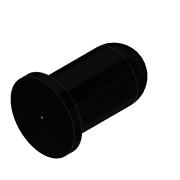
# Autodesk Inventor part: Photodiodendummie
Saved by Autodesk Inventor 2018.2 (Build 222227000, 227)
## iProperties
Created: 2018-10-30
Part Number: Photodiodendummie
Material: Kst - PEEK GF30
Document SubType Name: Modeling
Designer: N.Grubert
Density: 1.49 g/cm^3
Appearance: Grau (Schiefer)
Fläche: 0 cm²
Gewicht: 0 g
Material: geeigneten Werkstoff auswählen !
Dateiname: P:\INVENTOR\Inventor 2018\Templates\ILT\Norm.ipt
Bez_eng: bolt
Bez_french: boulon
Author: N.Grubert
Autodesk Inventor part; units mm, degrees
ref_plane "YZ Plane" through (0, 0, 0) normal (1, 0, 0) x (0, 1, 0)
ref_plane "XZ Plane" through (0, 0, 0) normal (0, 1, 0) x (-1, 0, 0)
ref_plane "XY Plane" through (0, 0, 0) normal (0, 0, 1) x (1, 0, 0)
sketch "Skizze4" plane through (0, 0, 0) normal (1, 0, 0) x (0, 1, 0)
  line L0 (-1.2621, 0) -> (7.5728, 0) projected
  line L1 (0, 0) -> (0, 2)
  line L2 (0.5, 1.5) -> (4.5, 1.5)
  arc A0 (6, 0) -> (4.5, 1.5) centre (4.5, 0) ccw
  line L3 (0, 0) -> (6, 0)
  line L4 (0, -0.4) -> (0, 2.4) construction
  line L5 (0.5, 1.5) -> (0.5, 2)
  line L6 (0.5, 2) -> (0, 2)
  dimension "d4" = 3
  dimension "d5" = 6
  dimension "d7" = 0.5
  dimension "d8" = 0.5
  constraints: 10 end point, 2 collinear, 2 perpendicular, 2 point on circle, 2 point on line, 1 centre point, 1 line through centre, 1 tangent, 1 vertical
  measures "d4" diameter of L2 L0
  measures "d5" distance from line of L3.end L1
  measures "d7" distance between parallel lines of L6 L2
  measures "d8" distance of L5.end L1.end
revolve "Umdrehung1" add sketch "Skizze4" angle 360 about axis through (0, -10, 0) along (0, 1, 0)
equation "\"d7\" = d8"
